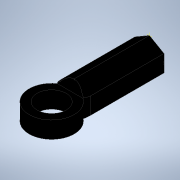
# Autodesk Inventor part: Cabezal
Saved by Autodesk Inventor 2020 (Build 240168000, 168)
## iProperties
Created: 2019-09-24
Part Number: Cabezal
Material: Plástico ABS
Document SubType Name: Modeling
Designer: Frederich Schnëider
Density: 1.06 g/cm^3
Appearance: Anodizado - Negro
Author: Frederich Schnëider
Autodesk Inventor part; units mm, degrees
sketch "Boceto1" plane through (0, 0, 0) normal (0, 0, 1) x (1, 0, 0)
  line L0 (2.7452, 1.596) -> (2.7548, -1.5794)
  line L1 (2.7548, -1.5794) -> (0.0096, -3.1754)
  line L2 (0.0096, -3.1754) -> (-2.7452, -1.596)
  line L3 (-2.7452, -1.596) -> (-2.7548, 1.5794)
  line L4 (-2.7548, 1.5794) -> (-0.0096, 3.1754)
  line L5 (-0.0096, 3.1754) -> (2.7452, 1.596)
  point P0 (0, 0)
  point P1 (0, 0)
  dimension "d0" = 5.5
  dimension "d20" = 6.3508
  constraints: 12 end point, 1 coincident, 3 other
  measures "d0" distance between parallel lines of L0 L3
  measures "d20" vertical distance of L4.end L1.end
extrude "Extrusión1" add sketch "Boceto1" along normal blind 15
ref_plane "Plano de trabajo4" through (-2.7452, -1.596, 0) normal (0, 0, -1) x (-1, 0, 0)
sketch "Boceto2" plane through (-2.7452, -1.596, 0) normal (0, 0, -1) x (-1, 0, 0)
  line L0 (-2.7548, -1.5794) -> (1.0358, -1.5794)
  line L1 (1.0358, -1.5794) -> (-2.7548, -1.5794)
  line L2 (-5.6299, -1.5794) -> (-2.7548, -1.5794)
  point P0 (-2.7452, 1.596)
  dimension "d5" = 3.1754
  constraints: 6 end point, 2 horizontal, 1 collinear, 1 point on line
  measures "d5" distance of L0.start point (-2.745, 1.596)
ref_plane "Plano de trabajo5" through (0, -3.175, 0) normal (0, 1, 0) x (-1, 0, 0)
sketch "Boceto3" plane through (0, -3.175, 0) normal (0, 1, 0) x (-1, 0, 0)
  line L0 (-0.0096, 15) -> (-2.7548, 15) projected
  line L1 (2.6199, 14) -> (-2.7548, 14) construction
  line L2 (-0.0096, 0) -> (-0.0096, 15) projected
  line L3 (-0.0096, 14) -> (-0.0096, 18.5)
  circle A0 centre (-0.0096, 18.5) radius 4.25
  circle A1 centre (-0.0096, 18.5) radius 2.75
  point P0 (0, 0)
  dimension "d7" = 1
  dimension "d8" = 4.5
  dimension "d9" = 8.5
  dimension "d14" = 5.5
  constraints: 4 end point, 2 centre point, 2 coincident, 2 point on line, 1 collinear, 1 horizontal
  measures "d7" distance between parallel lines of L1 L0
  measures "d8" distance of L3.start L3.end
  measures "d9" diameter of A0
  measures "d14" diameter of A1
sketch "Boceto4" plane through (-2.7452, -1.596, 0) normal (0, 0, -1) x (-1, 0, 0)
  point P0 (-2.7452, 1.596)
  point P1 (-2.7356, 4.7714)
  point P2 (-2.7548, -1.579)
  dimension "d10" = 6.3504
  measures "d10" vertical distance of point (-2.755, -1.579) point (-2.736, 4.771)
extrude "Extrusión2" add sketch "Boceto3" along normal blind 6.35 contours L2 A0 L0 | L0 A0 L2 | A1
ref_plane "Barreno" through (0, 0, 0) normal (0, -1, 0) x (1, 0, 0)
sketch "Boceto6" plane through (0, 0, 0) normal (0, -1, 0) x (1, 0, 0)
  arc A0 (0.0103, 14.25) -> (0.0089, 14.25) centre (0.0096, 18.5) ccw projected
  circle A1 centre (0.0096, 18.5) radius 2.75 projected
  point P0 (0, 0)
  dimension "d13" = 4.25
  measures "d13" radius of A0
extrude "Extrusión3" cut sketch "Boceto6" along normal mid plane 10 contours A1
ref_plane "Plano de trabajo8" through (5, 0, 0) normal (1, 0, 0) x (0, 1, 0)
sketch "Boceto8" plane through (5, 0, 0) normal (1, 0, 0) x (0, 1, 0)
  line L0 (-3.175, 15.75) -> (-3.175, 21.25) projected
  line L1 (-3.1754, 14.25) -> (-1.5794, 15)
  line L2 (-1.5794, 15) -> (-1.5794, 22.75)
  line L3 (-1.5794, 22.75) -> (-3.175, 22.75)
  line L4 (3.175, 14.25) -> (1.596, 15)
  line L5 (1.596, 15) -> (1.596, 22.75)
  line L6 (1.596, 22.75) -> (3.175, 22.75)
  ellipse E0 centre (3.1866, 18.5) end of major axis (3.1866, 14.25) minor radius 2.4709 (1.7849, 15) -> (3.175, 14.25) ccw projected
  line L7 (-3.175, 22.75) -> (-6.1952, 22.75)
  line L8 (-6.1952, 22.75) -> (-6.1952, 14.0055)
  line L9 (-6.1952, 14.0055) -> (-3.1754, 14.25)
  line L10 (3.175, 14.25) -> (7.2865, 13.4418)
  line L11 (7.2865, 13.4418) -> (6.5328, 22.75)
  line L12 (6.5328, 22.75) -> (3.175, 22.75)
  point P0 (0, 0)
  point P1 (-1.5794, 15)
  constraints: 24 end point, 5 perpendicular, 2 coincident, 2 point on line, 1 horizontal, 1 vertical, 1 other
extrude "Extrusión4" cut sketch "Boceto8" against normal blind 10 contours L9 L8 L7 L3 L2 L1 | L4 L5 L6 L12 L11 L10
fillet "Empalme1" radius 2 1 edges at (-2.75, 0, 15)
fillet "Empalme2" radius 2 1 edges at (2.75, 0.0083, 15)
ref_plane "Plano de trabajo9" through (0, 0, 0) normal (0, 0, -1) x (-1, 0, 0)
sketch "Boceto9" plane through (0, 0, 0) normal (0, 0, -1) x (-1, 0, 0)
  circle A0 centre (0, 0) radius 2.75
  line L0 (2.7548, 1.5794) -> (2.7452, -1.596) projected
  constraints: 1 centre point, 1 coincident, 1 tangent
extrude "Extrusión5" add sketch "Boceto9" along normal blind 0.01
